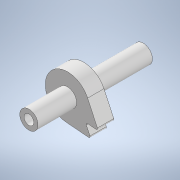
# Autodesk Inventor part: reverser-base
Saved by Autodesk Inventor 2021 (Build 250183000, 183)
## iProperties
Created: 2021-07-09
Part Number: reverser-base
Material: Generic
Document SubType Name: Modeling
Designer: teh18
Density: 1 g/cm^3
Appearance: Default
Author: teh18
Autodesk Inventor part; units mm, degrees
ref_plane "YZ Plane" through (0, 0, 0) normal (1, 0, 0) x (0, 1, 0)
ref_plane "XZ Plane" through (0, 0, 0) normal (0, 1, 0) x (-1, 0, 0)
ref_plane "XY Plane" through (0, 0, 0) normal (0, 0, 1) x (1, 0, 0)
sketch "Sketch1" plane through (0, 0, 0) normal (0, 0, 1) x (1, 0, 0)
  line L0 (2.6, -0.6) -> (-2.6, -0.6) projected
  line L1 (-2.6, -0.6) -> (-2.6, 0.6) projected
  line L2 (-2.6, 0.6) -> (2.6, 0.6) projected
  line L3 (2.6, 0.6) -> (2.6, -0.6) projected
  circle A0 centre (0, 0) radius 3.6 projected
  line L4 (-2.7, 0.7) -> (-2.7, -0.7)
  line L5 (-2.7, -0.7) -> (2.7, -0.7)
  line L6 (2.7, -0.7) -> (2.7, 0.7)
  line L7 (2.7, 0.7) -> (-2.7, 0.7)
  circle A1 centre (0, 0) radius 5.6
  dimension "d0" = 0.1
  dimension "d5" = 2
  constraints: 8 end point, 1 centre point, 3 other
  measures "d0" distance between parallel lines of L1 L4
  measures "d5" radial gap between concentric circles of A0 A1
extrude "Extrusion1" add sketch "Sketch1" along normal blind 10 contours A0 | A1
sketch "Sketch2" plane through (0, 0, 10) normal (0, 0, 1) x (0, -1, 0)
  line L0 (-0.7, -2.7) -> (-0.7, 2.7) projected
  line L1 (-0.7, 2.7) -> (0.7, 2.7) projected
  line L2 (0.7, 2.7) -> (0.7, -2.7) projected
  line L3 (0.7, -2.7) -> (-0.7, -2.7) projected
  circle A0 centre (0, 0) radius 3.75
  circle A1 centre (0, 0) radius 5.6 projected
  constraints: 1 centre point, 2 other
ref_plane "Work Plane1" through (-14, -11, 93) normal (0, 0, -1) x (0, 1, 0)
extrude "Extrusion2" add sketch "Sketch2" along normal blind 60 contours L0 L1 L2 L3 | A0 | A1
ref_plane "Work Plane2" through (0, 0, 36.375) normal (0, 0, -1) x (-1, 0, 0)
sketch "Sketch4" plane through (0, 0, 70) normal (0, 0, 1) x (1, 0, 0)
  circle A0 centre (0, 0) radius 3
  dimension "d20" = 6
  constraints: 1 centre point, 1 coincident
  measures "d20" diameter of A0
extrude "Extrusion4" cut sketch "Sketch4" against normal blind 10
sketch "Sketch5" plane through (0, 0, 60) normal (0, 0, 1) x (1, 0, 0)
  circle A0 centre (0, 0) radius 3 projected
  circle A1 centre (0, 0) radius 3 projected
  line L0 (-3, 0.5) -> (3, 0.5)
  line L1 (3, 0.5) -> (3, -0.5)
  line L2 (3, -0.5) -> (-3, -0.5)
  line L3 (-3, -0.5) -> (-3, 0.5)
  line L4 (-3, 0.5) -> (3, -0.5) construction
  line L5 (3, 0.5) -> (-3, -0.5) construction
  point P0 (-2.958, -0.5)
  point P1 (2.958, -0.5)
  point P2 (2.958, 0.5)
  point P3 (-2.958, 0.5)
  dimension "d24" = 6
  dimension "d25" = 1
  constraints: 12 end point, 2 midpoint, 2 parallel, 1 horizontal, 1 perpendicular
  measures "d24" distance of L1.end L2.end
  measures "d25" distance of L0.end L1.end
extrude "Extrusion5" add sketch "Sketch5" along normal blind 0.8 contours A0 L2 L0
sketch "Sketch6" plane through (0, 0, 36.375) normal (0, 0, -1) x (-1, 0, 0)
  circle A0 centre (0, 0) radius 5.6 projected
  circle A1 centre (0, 0) radius 13.6
  circle A2 centre (-67.3725, -47) radius 18
  circle A3 centre (-67.3725, -47) radius 38
  circle A4 centre (-67.3725, -47) radius 50
  line L0 (1.1617, -13.5503) -> (-14.3417, -14.8794)
  line L1 (-12.3158, 5.7691) -> (-18.9164, -8.3218)
  line L2 (0, 0) -> (-26.365, -18.3926)
  line L3 (-14.3417, -14.8794) -> (-10.9499, -7.6388)
  line L4 (-10.9499, -7.6388) -> (-18.9164, -8.3218)
  circle A5 centre (-67.3725, -47) radius 62
  line L5 (7.7812, -11.154) -> (-14.8595, -26.9486)
  line L6 (-12.3158, 5.7691) -> (-35.4273, -10.3539)
  point P0 (-11.2354, -7.6633)
  point P1 (-11.0715, -7.8983)
  dimension "d30" = 8
  dimension "d34" = 60
  dimension "d35" = 12
  dimension "d36" = 30
  dimension "d37" = 30
  constraints: 14 end point, 5 point on circle, 4 centre point, 3 tangent, 2 parallel, 1 coincident, 1 point on line, 7 other
  measures "d30" radial gap between concentric circles of A0 A1
  measures "d34" angle of L3 L0
  measures "d36" angle of L0 L5
  measures "d37" angle of L6 L1
extrude "Extrusion6" add sketch "Sketch6" against normal blind 10 contours A1 L3 L4 | A1 L4 L1 | L4 L2 A1 | L0 L3 A1 | L2 L3 A1
fillet "Fillet1" radius 0.8 4 edges at (14.3417, -14.8794, 41.375) (18.9164, -8.3218, 41.375) (11.0715, -7.8983, 41.375) (11.2354, -7.6633, 41.375)
equation "\"d37\" = d36"
body "Solid1"
